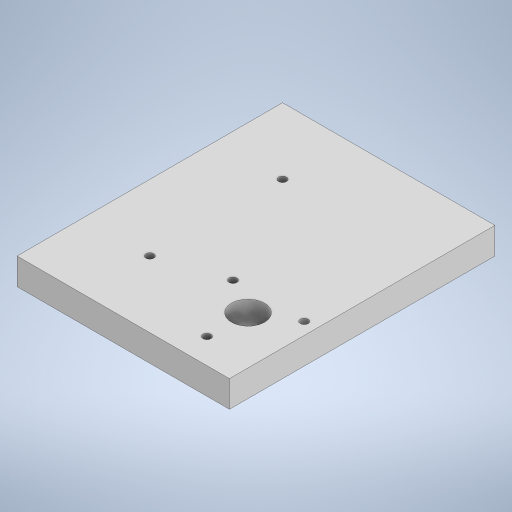
# Autodesk Inventor part: Support test1
Saved by Autodesk Inventor 2024.2 (Build 282272000, 272)
## iProperties
Created: 2024-03-08
Part Number: Support test1
Material: Generic
Document SubType Name: Modeling
Designer: evmgm
Density: 1 g/cm^3
Appearance: Default
Author: evmgm
Autodesk Inventor part; units mm, degrees
ref_plane "YZ Plane" through (0, 0, 0) normal (1, 0, 0) x (0, 1, 0)
ref_plane "XZ Plane" through (0, 0, 0) normal (0, 1, 0) x (-1, 0, 0)
ref_plane "XY Plane" through (0, 0, 0) normal (0, 0, 1) x (1, 0, 0)
sketch "Sketch1" plane through (0, 0, 0) normal (0, 1, 0) x (-1, 0, 0)
  line L0 (0, 0) -> (80, 0)
  line L1 (80, 0) -> (80, -100)
  line L2 (80, -100) -> (0, -100)
  line L3 (0, -100) -> (0, 0)
  line L4 (55, 12.5326) -> (55, -107.8943) construction
  circle A0 centre (55, -25) radius 1.5
  circle A1 centre (55, -75) radius 1.5
  line L5 (55, -25) -> (18, -25) construction
  circle A2 centre (18, -25) radius 1.5
  circle A3 centre (18, -25) radius 6.25
  circle A4 centre (18, -9.5) radius 1.5
  circle A5 centre (4.5766, -32.75) radius 1.5
  circle A6 centre (31.4234, -32.75) radius 1.5
  dimension "d2" = 25
  dimension "d3" = 3
  dimension "d4" = 3
  dimension "d5" = 25
  dimension "d6" = 50
  dimension "d7" = 37
  dimension "d8" = 3
  dimension "d9" = 100
  dimension "d10" = 80
  dimension "d13" = 12.5
  dimension "d16" = 3
  dimension "d17" = 15.5
  dimension "d20" = 360
  dimension "d22" = 12.5326
  dimension "d23" = 107.8943
  dimension "d27" = 48.5766
  constraints: 12 end point, 7 centre point, 4 coincident, 2 horizontal, 2 parallel, 2 point on line, 1 perpendicular, 1 vertical, 8 other
  measures "d2" distance between parallel lines of L1 L4
  measures "d3" diameter of A0
  measures "d4" diameter of A1
  measures "d5" distance from line of L0 L5.start
  measures "d6" distance of L5.start A1.centre
  measures "d7" distance of L5.start L5.end
  measures "d8" diameter of A2
  measures "d9" distance of L0.end L1.end
  measures "d10" distance between parallel lines of L1 L3
  measures "d13" diameter of A3
  measures "d16" diameter of A4
  measures "d17" distance of L5.end A4.centre
  measures "d22" distance from line of L4.start L0
  measures "d23" distance from line of L4.end L0
  measures "d27" distance from line of A6.centre L1
extrude "Extrusion1" add sketch "Sketch1" along normal blind 10 contours L0 L1 L2 L3 | A3 | A4 | A5 | A6
extrude "Extrusion2" cut sketch "Sketch1" along normal blind 10 contours A3
extrude "Extrusion3" cut sketch "Sketch1" along normal blind 10 contours A4 | A5 | A6
body "Solid1"
